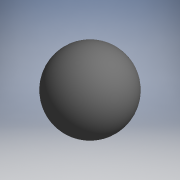
# Autodesk Inventor part: MR126ZZ Ball
Saved by Autodesk Inventor 2017.3 (Build 213256000, 256)
## iProperties
Part Number: MR126ZZ Ball
Material: Generic
Catalog Web Link: www.cadenas.de
Description: shielde_type_zz_zzs_B-
Vendor: NSK_RB
Document SubType Name: Modeling
Designer: partserver
Manufacturer: NSK_RB
Mass: 0.00305363 g
Surface Area: 0.101788 cm^2
Volume: 0.00305363 cm^3
Density: 1 g/cm^3
Appearance: PSOLRGB-128-128-128
Category: PARTsolutions
Company: NSK_RB
Title: MR126ZZ Ball
Author: Cadenas PARTsolutions
PSOL_IDENT_0: {$CADENAS_DATA\23d-libs\nsk_rb\roller_bearings\deep_groove_bb\exstra_small_miniatur_bb\metric_design
PSOL_IDENT_1: \shielded_type_zz_zzs_b.prj},180 {VTYP=3D},{NB=MR126ZZ Ball},{LINA=MR126ZZ Ball},{NN=shielde_type_zz
PSOL_IDENT_2: _zzs_B},{DATE=16.07.2021 00:25:30},{GEOMDATE=04.01.2008 00:00:00},{VERSION=},{LINEID=590},{WBVAR=},{
PSOL_IDENT_3: WBNUMERIC=}  {NB=MR126ZZ Ball},{LINA=MR126ZZ Ball},{KT=DUMMY},{IDNR=},{STAN=Standard},{ORDER=MR126ZZ
PSOL_IDENT_4: },{SD=6.0},{X=6.0},{DI1=7.73},{DI2=7.20},{SDE1=10.19},{SDE2=10.90},{D=12},{DD=12},{B=0.0},{B1=4.0},{
PSOL_IDENT_5: R=0.00},{R1=0.15},{CR1=715},{COR1=292},{CR2=73},{COR2=30.0},{LG=43000},{LO=50000},{DA=0.0},{DB=7.2},
PSOL_IDENT_6: {DA1=0.0},{DB1=10.9},{RA=0.00},{RB=0.15},{MASS=1.74},{SC=1}
NB: MR126ZZ Ball
NN: shielde_type_zz_zzs_B
NBSYN: $ORDER. Ball
LINA: MR126ZZ Ball
CATALOG: NSK Rolling Bearing
STAN: Standard
ORDER: MR126ZZ
SD: 6
X: 6
DI1: 7.73
DI2: 7.2
SDE1: 10.19
SDE2: 10.9
D: 12
DD: 12
B: 0
B1: 4
R: 0
R1: 0.15
CR1: 715
COR1: 292
CR2: 73
COR2: 30
LG: 43000
LO: 50000
DA: 0
DB: 7.2
DA1: 0
DB1: 10.9
RA: 0
RB: 0.15
MASS: 1.74
SC: 1
SUPPLIER: NSK_RB
ARTICLENO: MR126ZZ Ball
BOMINFO: MR126ZZ Ball
CREATOR: CADENAS GmbH
Autodesk Inventor part; units mm, degrees
sketch "Sketch_1" plane through (0, 0, 0) normal (0, 0, 1) x (1, 0, 0)
  line L0 (0.9, 0) -> (-0.9, 0)
  arc A0 (0.9, 0) -> (-0.9, 0) centre (0, 0) ccw
  line L1 (0.9, 0) -> (-0.9, 0)
  constraints: 4 end point, 2 point on circle, 1 centre point
revolve "Revolution1" add sketch "Sketch_1" angle 360 about axis through (0.9, 0, 0) along (1, 0, 0)
ref_plane "ip_st_b_XY" through (0, 0, 0) normal (-1, 0, 0) x (0, 0, -1)
ref_plane "ip_st_b_YZ" through (0, 0, 0) normal (0, 0, -1) x (0, -1, 0)
ref_plane "ip_st_b_ZX" through (0, 0, 0) normal (0, -1, 0) x (-1, 0, 0)
body "Solid1"
